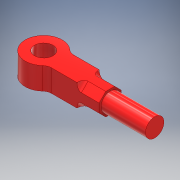
# Autodesk Inventor part: Eye end
Saved by Autodesk Inventor 2018 (Build 220112000, 112)
## iProperties
Created: 2020-01-29
Part Number: Eye end
Material: Plástico PC/ABS
Document SubType Name: Modeling
Designer: aidan
Density: 0.357273 g/cm^3
Appearance: Suave - Blanco
Author: aidan
Autodesk Inventor part; units mm, degrees
ref_plane "YZ Plane" through (0, 0, 0) normal (1, 0, 0) x (0, 1, 0)
ref_plane "XZ Plane" through (0, 0, 0) normal (0, 1, 0) x (-1, 0, 0)
ref_plane "XY Plane" through (0, 0, 0) normal (0, 0, 1) x (1, 0, 0)
sketch "Boceto1" plane through (0, 0, 0) normal (0, 0, 1) x (1, 0, 0)
  arc A0 (33.9935, 36.6667) -> (33.9935, -36.6667) centre (0, 0) ccw
  circle A1 centre (0, 0) radius 25
  line L0 (50.9902, 30) -> (180, 30)
  line L1 (180, 30) -> (180, -30)
  line L2 (180, -30) -> (50.9902, -30)
  arc A2 (33.9935, 36.6667) -> (50.9902, 30) centre (50.9902, 55) ccw
  arc A3 (50.9902, -30) -> (33.9935, -36.6667) centre (50.9902, -55) ccw
  dimension "d0" = 100
  dimension "d1" = 50
  dimension "d6" = 50
  dimension "d7" = 50
  constraints: 6 end point, 6 point on circle, 4 centre point, 4 tangent, 2 coincident, 1 horizontal, 1 parallel, 1 perpendicular
  measures "d0" diameter of A0
  measures "d1" diameter of A1
  measures "d6" diameter of A2
  measures "d7" diameter of A3
extrude "Extrusión1" add sketch "Boceto1" along normal blind 60
sketch "Boceto2" plane through (180, -30, 0) normal (1, 0, 0) x (0, 0, -1)
  line L0 (0, 60) -> (-60, 60) projected
  line L1 (0, 0) -> (0, 60) projected
  line L2 (0, 60) -> (-18.06, 60)
  line L3 (0, 60) -> (0, 41.94)
  line L4 (0, 80) -> (0, -20) projected
  line L5 (0, 41.94) -> (-18.06, 60)
  line L6 (-41.94, 60) -> (-60, 41.94)
  line L7 (-60, 60) -> (-60, 41.94)
  line L8 (-60, 60) -> (-41.94, 60)
  line L9 (-60, 18.06) -> (-41.94, 0)
  line L10 (-60, 0) -> (-41.94, 0)
  line L11 (-60, 0) -> (-60, 18.06)
  line L12 (-18.06, 0) -> (0, 18.06)
  line L13 (0, 0) -> (0, 18.06)
  line L14 (0, 0) -> (-18.06, 0)
  point P0 (0, 30)
  point P1 (-30, 30)
  point P2 (-30, 60)
  point P3 (0, 30)
  point P4 (0, 66.6667)
  point P5 (0, -6.6667)
  dimension "d11" = 18.06
  dimension "d12" = 18.06
  dimension "d15" = 360
  constraints: 24 end point, 2 midpoint, 1 horizontal alignment, 1 point on line, 1 vertical alignment, 27 other
  measures "d11" distance of L0.start L2.end
  measures "d12" distance of L0.start L3.end
extrude "Extrusión3" cut sketch "Boceto2" against normal blind 60
sketch "Boceto3" plane through (180, -11.94, 0) normal (1, 0, 0) x (0, 0, -1)
  circle A0 centre (-30, 11.94) radius 25
  line L0 (-18.06, 41.94) -> (-41.94, 41.94) projected
  line L1 (0, 0) -> (0, 23.88) projected
  point P0 (0, 11.94)
  point P1 (-30, 41.94)
  point P2 (0, 11.94)
  dimension "d21" = 50
  constraints: 2 midpoint, 1 centre point, 1 horizontal alignment, 1 vertical alignment
  measures "d21" diameter of A0
extrude "Extrusión4" add sketch "Boceto3" along normal blind 120.5
fillet "Empalme1" radius 12 4 edges at (120, 20.97, 50.97) (120, 20.97, 9.03) (120, -20.97, 9.03) (120, -20.97, 50.97)
